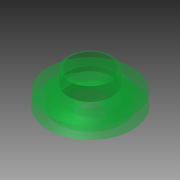
# Autodesk Inventor part: Suctin Cup Part 1 1764
Saved by Autodesk Inventor 2011 (Build 150239000, 239)
## iProperties
Created: 2010-02-08
Part Number: Suctin Cup Part 1 1764
Document SubType Name: Modeling
Designer: clee1
Density: 1 g/cm^3
Author: clee1
Autodesk Inventor part; units mm, degrees
ref_plane "YZ Plane" through (0, 0, 0) normal (1, 0, 0) x (0, 1, 0)
ref_plane "XY Plane" through (0, 0, 0) normal (0, 0, 1) x (1, 0, 0)
sketch "Sketch1" plane through (0, 0, 0) normal (0, 0, 1) x (1, 0, 0)
  line L0 (-43.0614, 14.0592) -> (-55.1736, 10.2402)
  line L1 (-55.1736, 10.2402) -> (-43.0614, 6.4212)
  line L2 (-43.0614, 6.4212) -> (-55.1736, 2.6023)
  line L3 (-55.1736, 2.6023) -> (-43.0614, -1.2167)
  line L4 (-43.0614, 14.0592) -> (-43.0614, 22.3142)
  line L5 (-41.2446, 22.887) -> (-41.2446, 12.727)
  line L6 (-41.2446, 12.727) -> (-49.1317, 10.2402)
  line L7 (-49.1317, 10.2402) -> (-37.0195, 6.4212)
  line L8 (-37.0195, 6.4212) -> (-49.1317, 2.6023)
  line L9 (-49.1317, 2.6023) -> (-37.0195, -1.2167)
  line L10 (-41.2446, 22.887) -> (-43.0614, 22.3142)
  line L11 (-29.7736, 28.5538) -> (-29.7736, -8.0637)
  line L12 (8.7272, 15.7537) -> (-3.385, 11.9347)
  line L13 (14.7691, 15.7537) -> (-2.8387, 10.202)
  line L14 (-2.8387, 10.202) -> (-3.385, 11.9347)
  line L15 (14.7691, 15.7537) -> (8.7272, 15.7537)
  line L16 (-37.0195, -1.2167) -> (-43.0614, -1.2167)
  point P0 (0, 0)
  dimension "d1" = 12.7
  dimension "d2" = 12.7
  dimension "d3" = 8.255
  dimension "d4" = 1.905
  dimension "d7" = 25.4
  constraints: 34 end point, 6 parallel, 2 equal length, 1 perpendicular, 1 point on line, 1 vertical, 4 other
  measures "d1" distance of L0.start L0.end
  measures "d2" distance of L0.end L1.end
  measures "d3" distance of L0.start L4.end
  measures "d4" distance of L5.start L4.end
  measures "d7" distance from line of L0.end L11
revolve "Revolution1" add sketch "Sketch1" angle 360 about axis through (-29.7736, 28.5538, 0) along (0, -1, 0) contours L4 L10 L5 L6 L7 L8 L9 L16 L3 L2 L1 L0
ref_plane "Work Plane1" through (0, 23.8125, 0) normal (0, 1, 0) x (-1, 0, 0)
body "Solid1"
